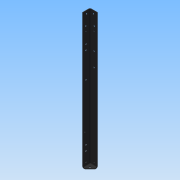
# Autodesk Inventor part: стойка
Saved by Autodesk Inventor 2017 (Build 210142000, 142)
## iProperties
Part Number: стойка
Material: Типовые
Document SubType Name: Modeling
Designer: Max
Mass: 21.5367 g
Surface Area: 277.328 cm^2
Volume: 21.5367 cm^3
Density: 1 g/cm^3
Appearance: Резина — черная
Author: Max
Autodesk Inventor part; units mm, degrees
ref_plane "YZ Plane" through (0, 0, 0) normal (1, 0, 0) x (0, 1, 0)
ref_plane "XZ Plane" through (0, 0, 0) normal (0, 1, 0) x (-1, 0, 0)
ref_plane "XY Plane" through (0, 0, 0) normal (0, 0, 1) x (1, 0, 0)
sketch "Эскиз1" plane through (0, 0, 0) normal (0, 0, 1) x (1, 0, 0)
  line L0 (-236.7799, 208.2081) -> (-236.7799, 188.2081)
  line L1 (-216.7799, 208.2081) -> (-236.7799, 208.2081)
  line L2 (-236.7799, 188.2081) -> (-235.1299, 188.2081)
  line L3 (-235.1299, 188.2081) -> (-235.1299, 206.5581)
  line L4 (-235.1299, 206.5581) -> (-216.7799, 206.5581)
  line L5 (-216.7799, 206.5581) -> (-216.7799, 208.2081)
  line L6 (-216.7799, 206.5581) -> (-216.7799, 201.4081)
  line L7 (-216.7799, 201.4081) -> (-229.9799, 188.2081)
  line L8 (-229.9799, 188.2081) -> (-235.1299, 188.2081)
  line L9 (-236.7799, 208.2081) -> (-223.3799, 194.8081) construction
  circle A0 centre (-226.7799, 198.2081) radius 2
  point P0 (0, 0)
  dimension "d0" = 20
  dimension "d1" = 20
  dimension "d2" = 1.65
  dimension "d3" = 1.65
  dimension "d6" = 6.8
  dimension "d7" = 6.8
  dimension "d10" = 4
  dimension "d11" = 10
  constraints: 20 end point, 5 perpendicular, 2 vertical, 1 centre point, 1 horizontal, 1 midpoint, 1 point on line
  measures "d0" distance of L1.start L0.start
  measures "d1" distance of L0.start L0.end
  measures "d2" distance of L0.end L2.end
  measures "d3" distance between parallel lines of L1 L4
  measures "d6" distance of L7.end L0.end
  measures "d7" distance from line of L6.end L1
  measures "d10" diameter of A0
  measures "d11" distance from line of L0 A0.centre
extrude "Выдавливание1" add sketch "Эскиз1" along normal blind 353 contours L1 L5 L4 L3 L2 L0
extrude "Выдавливание2" add sketch "Эскиз1" along normal blind 1.65 contours L3 L4 L6 L7 L8 | A0
extrude "Выдавливание3" cut sketch "Эскиз1" along normal blind 1.65 contours A0
fillet "Сопряжение1" radius 2 1 edges at (-235.1299, 206.5581, 177.325)
fillet "Сопряжение2" radius 3.65 1 edges at (-236.7799, 208.2081, 176.5)
fillet "Сопряжение3" radius 3.65 3 edges at (-235.7109, 207.1391, 0) (-236.7799, 196.3831, 0) (-224.9549, 208.2081, 0)
fillet "Сопряжение4" radius 2 3 edges at (-234.5442, 205.9724, 1.65) (-235.1299, 196.3831, 1.65) (-224.9549, 206.5581, 1.65)
sketch "Эскиз2" plane through (-236.7799, 188.2081, 353) normal (-1, 0, 0) x (0, 0, 1)
  circle A0 centre (-344, 8.5) radius 1.5
  line L0 (-353, 16.35) -> (-353, 0) projected
  line L1 (-349.35, 0) -> (0, 0) projected
  circle A1 centre (-318.5, 8.5) radius 2
  circle A2 centre (-304.5, 8.5) radius 2
  line L2 (-318.5, 8.5) -> (-304.5, 8.5) construction
  circle A3 centre (-274, 5.5) radius 1.5
  circle A4 centre (-157, 8.5) radius 2
  circle A5 centre (-90, 8.5) radius 2
  circle A6 centre (-76, 8.5) radius 2
  line L3 (0, 16.35) -> (0, 0) projected
  circle A7 centre (-47, 8.5) radius 1.5
  circle A8 centre (-35, 8) radius 2
  circle A9 centre (-8, 10) radius 2
  point P0 (-353, -188.2081)
  dimension "d18" = 3
  dimension "d19" = 9
  dimension "d20" = 8.5
  dimension "d21" = 4
  dimension "d22" = 4
  dimension "d23" = 34.5
  dimension "d24" = 8.5
  dimension "d25" = 14
  dimension "d26" = 3
  dimension "d27" = 5.5
  dimension "d28" = 79
  dimension "d29" = 4
  dimension "d30" = 8.5
  dimension "d31" = 196
  dimension "d32" = 4
  dimension "d33" = 4
  dimension "d34" = 8.5
  dimension "d35" = 8.5
  dimension "d36" = 90
  dimension "d37" = 14
  dimension "d38" = 3
  dimension "d39" = 8.5
  dimension "d40" = 47
  dimension "d41" = 4
  dimension "d42" = 4
  dimension "d43" = 8
  dimension "d44" = 10
  dimension "d45" = 8
  dimension "d46" = 27
  dimension "d47" = 12
  constraints: 10 centre point, 2 end point, 1 horizontal
  measures "d18" diameter of A0
  measures "d19" distance from line of A0.centre L0
  measures "d20" distance from line of L1 A0.centre
  measures "d21" diameter of A1
  measures "d22" diameter of A2
  measures "d23" distance from line of L0 L2.start
  measures "d24" distance from line of L1 L2.start
  measures "d25" distance of L2.start L2.end
  measures "d26" diameter of A3
  measures "d27" distance from line of L1 A3.centre
  measures "d28" distance from line of L0 A3.centre
  measures "d29" diameter of A4
  measures "d30" distance from line of L1 A4.centre
  measures "d31" distance from line of L0 A4.centre
  measures "d32" diameter of A5
  measures "d33" diameter of A6
  measures "d34" distance from line of L1 A5.centre
  measures "d35" distance from line of L1 A6.centre
  measures "d36" distance from line of L3 A5.centre
  measures "d37" distance of A5.centre A6.centre
  measures "d38" diameter of A7
  measures "d39" distance from line of L1 A7.centre
  measures "d40" distance from line of L3 A7.centre
  measures "d41" diameter of A8
  measures "d42" diameter of A9
  measures "d43" distance from line of L1 A8.centre
  measures "d44" distance from line of L1 A9.centre
  measures "d45" distance from line of L3 A9.centre
  measures "d46" horizontal distance of A8.centre A9.centre
  measures "d47" horizontal distance of A8.centre A7.centre
extrude "Выдавливание4" cut sketch "Эскиз2" against normal blind 1.65
sketch "Эскиз3" plane through (-233.1299, 208.2081, 353) normal (0, 1, 0) x (1, 0, 0)
  circle A0 centre (7.85, 344) radius 1.5
  line L0 (16.35, 353) -> (0, 353) projected
  line L1 (16.35, 349.35) -> (16.35, 0) projected
  circle A1 centre (8.35, 35) radius 2
  circle A2 centre (6.35, 8) radius 2
  line L2 (16.35, 0) -> (0, 0) projected
  circle A3 centre (7.85, 47) radius 1.5
  circle A4 centre (7.85, 129) radius 2
  circle A5 centre (7.85, 92) radius 2
  point P0 (233.1299, 353)
  dimension "d50" = 3
  dimension "d51" = 9
  dimension "d52" = 8.5
  dimension "d53" = 4
  dimension "d54" = 4
  dimension "d55" = 8
  dimension "d56" = 10
  dimension "d57" = 27
  dimension "d58" = 8
  dimension "d59" = 3
  dimension "d60" = 8.5
  dimension "d61" = 12
  dimension "d62" = 4
  dimension "d63" = 4
  dimension "d64" = 8.5
  dimension "d65" = 8.5
  dimension "d66" = 37
  dimension "d67" = 92
  constraints: 6 centre point
  measures "d50" diameter of A0
  measures "d51" distance from line of L0 A0.centre
  measures "d52" distance from line of L1 A0.centre
  measures "d53" diameter of A1
  measures "d54" diameter of A2
  measures "d55" distance from line of L1 A1.centre
  measures "d56" distance from line of L1 A2.centre
  measures "d57" vertical distance of A1.centre A2.centre
  measures "d58" distance from line of L2 A2.centre
  measures "d59" diameter of A3
  measures "d60" distance from line of L1 A3.centre
  measures "d61" vertical distance of A1.centre A3.centre
  measures "d62" diameter of A4
  measures "d63" diameter of A5
  measures "d64" distance from line of L1 A5.centre
  measures "d65" distance from line of L1 A4.centre
  measures "d66" distance of A5.centre A4.centre
  measures "d67" distance from line of L2 A5.centre
extrude "Выдавливание5" cut sketch "Эскиз3" against normal blind 1.65
sketch "Эскиз4" plane through (-233.1299, 208.2081, 353) normal (0, 1, 0) x (1, 0, 0)
  line L0 (13.85, 9) -> (16.35, 9)
  line L1 (16.35, 349.35) -> (16.35, 0) projected
  line L2 (16.35, 9) -> (16.35, 16)
  line L3 (16.35, 16) -> (13.85, 16)
  arc A0 (13.85, 16) -> (13.85, 9) centre (13.85, 12.5) ccw
  line L4 (16.35, 0) -> (0, 0) projected
  point P0 (233.1299, 353)
  dimension "d72" = 3.5
  dimension "d73" = 7
  dimension "d74" = 6
  dimension "d75" = 9
  constraints: 6 end point, 2 point on circle, 1 centre point, 1 horizontal, 1 point on line, 1 tangent, 1 vertical
  measures "d72" radius of A0
  measures "d73" distance between parallel lines of L3 L0
  measures "d75" distance between parallel lines of L4 L0
extrude "Выдавливание6" cut sketch "Эскиз4" against normal blind 10
sketch "Эскиз5" plane through (-236.7799, 188.2081, 353) normal (-1, 0, 0) x (0, 0, 1)
  arc A0 (-9, 2.5) -> (-16, 2.5) centre (-12.5, 2.5) ccw
  line L0 (-9, 2.5) -> (-9, 0)
  line L1 (-349.35, 0) -> (0, 0) projected
  line L2 (-9, 0) -> (-16, 0)
  line L3 (-16, 0) -> (-16, 2.5)
  line L4 (0, 16.35) -> (0, 0) projected
  point P0 (-353, -188.2081)
  dimension "d78" = 7
  dimension "d79" = 6
  dimension "d80" = 9
  constraints: 6 end point, 2 point on circle, 2 point on line, 1 centre point, 1 tangent, 1 vertical
  measures "d78" diameter of A0
  measures "d80" distance between parallel lines of L4 L0
extrude "Выдавливание7" cut sketch "Эскиз5" against normal blind 10
